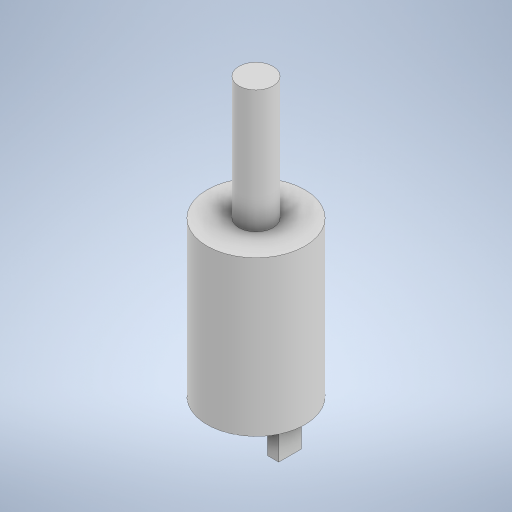
# Autodesk Inventor part: Dremel motor
Saved by Autodesk Inventor 2023 (Build 270158030, 158C)
## iProperties
Created: 2022-09-29
Part Number: Dremel motor
Material: Generic
Document SubType Name: Modeling
Designer: cjj5381
Density: 1 g/cm^3
Appearance: Default
Author: cjj5381
Autodesk Inventor part; units mm, degrees
ref_plane "YZ Plane" through (0, 0, 0) normal (1, 0, 0) x (0, 1, 0)
ref_plane "XZ Plane" through (0, 0, 0) normal (0, 1, 0) x (-1, 0, 0)
ref_plane "XY Plane" through (0, 0, 0) normal (0, 0, 1) x (1, 0, 0)
sketch "Sketch1" plane through (0, 0, 0) normal (0, 1, 0) x (-1, 0, 0)
  circle A0 centre (0, 0) radius 21.5
  dimension "d0" = 43
  constraints: 1 centre point, 1 coincident
  measures "d0" diameter of A0
extrude "Extrusion1" add sketch "Sketch1" along normal blind 68
sketch "Sketch2" plane through (0, 68, 0) normal (0, 1, 0) x (1, 0, 0)
  circle A0 centre (0, 0) radius 7.5
  dimension "d3" = 15
  constraints: 1 centre point, 1 coincident
  measures "d3" diameter of A0
extrude "Extrusion2" add sketch "Sketch2" along normal blind 54
sketch "Sketch3" plane through (0, 0, 0) normal (0, -1, 0) x (1, 0, 0)
  line L0 (-15, 5) -> (-10, 5)
  line L1 (-10, 5) -> (-10, -5)
  line L2 (-10, -5) -> (-15, -5)
  line L3 (-15, -5) -> (-15, 5)
  line L4 (10, 5) -> (15, 5)
  line L5 (15, 5) -> (15, -5)
  line L6 (15, -5) -> (10, -5)
  line L7 (10, -5) -> (10, 5)
  line L8 (0, 0) -> (-29.5746, 0)
  circle A0 centre (0, 0) radius 7.5 projected
  line L9 (0, 0) -> (0, 33.0968)
  dimension "d6" = 10
  dimension "d7" = 5
  dimension "d8" = 20
  constraints: 20 end point, 4 parallel, 3 horizontal, 3 symmetric about line, 2 perpendicular, 1 collinear, 1 point on line, 1 vertical
  measures "d6" distance of L4.end L5.end
  measures "d7" distance of L0.start L0.end
  measures "d8" distance of L0.end L4.start
extrude "Extrusion3" add sketch "Sketch3" along normal blind 15 contours L0 L1 L8 L3 | L8 L1 L2 L3 | L4 L5 L6 L7
body "Solid1"
